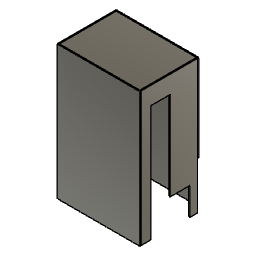
pc-case v8 (Autodesk Fusion 360 design; units mm, degrees)
Autodesk Fusion 360 part; units mm, degrees
sketch "Sketch1" plane through (0, 0, 0) normal (0, 1, 0) x (1, 0, 0) in component "Back"
  line L0 (0, 0) -> (210, 0)
  line L1 (210, 0) -> (210, -340)
  line L2 (210, -340) -> (0, -340)
  line L3 (0, -340) -> (0, 0)
  dimension "d1" = 210
  dimension "d2" = 340
  constraint horizontal L0
  constraint vertical L1
  constraint horizontal L2
  constraint vertical L3
  constraint coincident L0.start L3.end
  measures "d1" distance of L1.end L2.end
  measures "d2" distance of L0.start L2.end
extrude "Extrude1" add sketch "Sketch1" along normal blind 3 makes body 1 in component "Back"
sketch "Sketch1 (2)" plane through (0, 0, 0) normal (1, 0, 0) x (0, 1, 0) in component "right side"
  line L0 (2.986, 0.2323) -> (146.986, 0.2323)
  line L1 (146.986, 0.2323) -> (146.986, 310.2323)
  line L2 (146.986, 310.2323) -> (2.986, 310.2323)
  line L3 (2.986, 310.2323) -> (2.986, 0.2323)
  dimension "d5" = 310
  dimension "d6" = 144
  constraint horizontal L0
  constraint vertical L1
  constraint horizontal L2
  constraint vertical L3
  measures "d5" distance of L0.end L1.end
  measures "d6" distance of L0.start L0.end
extrude "Extrude1'" add sketch "Sketch1 (2)" along normal blind 3 separate body makes body 2 in component "right side"
sketch "Sketch1 (3)" plane through (0, 0, 0) normal (0, 0, 1) x (1, 0, 0) in component "top"
  line L0 (10, 145.6527) -> (214, 145.6527)
  line L1 (214, 145.6527) -> (214, 1.6527)
  line L2 (214, 1.6527) -> (10, 1.6527)
  line L3 (10, 1.6527) -> (10, 145.6527)
  dimension "d13" = 204
  dimension "d14" = 144
  constraint horizontal L0
  constraint vertical L1
  constraint horizontal L2
  constraint vertical L3
  measures "d13" distance of L0.start L0.end
  measures "d14" distance of L0.end L1.end
extrude "Extrude1''" add sketch "Sketch1 (3)" along normal blind 3 separate body makes body 3 in component "top"
sketch "Sketch1 (4)" plane through (0, 0, 0) normal (0, 1, 0) x (1, 0, 0) in component "front"
  line L0 (116.0218, -155.6494) -> (-93.9782, -155.6494)
  line L1 (-93.9782, -155.6494) -> (-93.9782, 169.3506)
  line L2 (-93.9782, 169.3506) -> (116.0218, 169.3506)
  line L3 (116.0218, 169.3506) -> (116.0218, -155.6494)
  dimension "d21" = 210
  dimension "d22" = 325
  constraint horizontal L0
  constraint vertical L1
  constraint horizontal L2
  constraint vertical L3
  measures "d21" distance of L0.start L0.end
  measures "d22" distance of L0.start L2.end
extrude "Extrude1'''" add sketch "Sketch1 (4)" along normal blind 3 separate body makes body 4 in component "front"
sketch "Sketch2" plane through (0, 0, 0) normal (1, 0, 0) x (0, 1, 0) in component "front"
sketch "Sketch1 (5)" plane through (0, 0, 0) normal (1, 0, 0) x (0, 1, 0) in component "left side"
  line L0 (-324, 340) -> (-180, 340)
  line L1 (-180, 340) -> (-180, 0)
  line L2 (-180, 0) -> (-200, 0)
  line L3 (-200, 0) -> (-200, 70)
  line L4 (-200, 70) -> (-250, 70)
  line L5 (-250, 70) -> (-250, 295)
  line L6 (-250, 295) -> (-299, 295)
  line L7 (-299, 295) -> (-299, 0)
  line L8 (-299, 0) -> (-324, 0)
  line L9 (-324, 0) -> (-324, 340)
  dimension "d29" = 144
  dimension "d30" = 340
  dimension "d31" = 295
  dimension "d32" = 25
  dimension "d33" = 20
  dimension "d34" = 70
  constraint horizontal L0
  constraint perpendicular L0 L1
  constraint perpendicular L1 L2
  constraint perpendicular L2 L3
  constraint perpendicular L1 L4
  constraint perpendicular L2 L5
  constraint perpendicular L5 L6
  constraint perpendicular L2 L7
  constraint perpendicular L7 L8
  constraint perpendicular L0 L9
  measures "d29" distance of L0.start L0.end
  measures "d30" distance of L0.end L1.end
  measures "d31" distance of L6.end L7.end
  measures "d32" distance of L7.end L8.end
  measures "d33" distance of L1.end L2.end
  measures "d34" distance of L2.end L3.end
extrude "Extrude1''''" add sketch "Sketch1 (5)" along normal blind 3 separate body makes body 5 in component "left side"
sketch "Sketch1 (6)" plane through (0, 0, 0) normal (0, 1, 0) x (1, 0, 0)
sketch "Sketch3" plane through (0, 3, 0) normal (0, 1, 0) x (-1, 0, 0) in component "front"
  line L0 (-116.0218, -169.3506) -> (93.9782, -169.3506)
  line L1 (93.9782, -169.3506) -> (93.9782, 155.6494)
  line L2 (93.9782, 155.6494) -> (-116.0218, 155.6494)
  line L3 (-116.0218, 155.6494) -> (-116.0218, -169.3506)
  line L4 (-116.0218, -169.3506) -> (-96.0218, -169.3506)
  line L5 (-96.0218, -169.3506) -> (-96.0218, -64.3506)
  line L6 (-96.0218, -64.3506) -> (-116.0218, -64.3506)
  line L7 (-116.0218, -64.3506) -> (-116.0218, -169.3506)
  dimension "d41" = 20
  dimension "d42" = 105
  constraint horizontal L4
  constraint vertical L5
  constraint horizontal L6
  constraint vertical L7
  constraint coincident L0.start L3.end
  measures "d41" distance of L5.end L6.end
  measures "d42" distance of L4.end L5.end
extrude "Extrude2" cut sketch "Sketch3" against normal blind 3 contours L0 L3 L4 L5 L6 L7 bodies 4 in component "front"
component "Back" placed x (1, 0, 0) y (0, 1, 0) z (0, 0, 1) at (7, -1.3473, -337)
component "right side" placed x (1, 0, 0) y (0, 1, 0) z (0, 0, 1) at (7, -1.3333, -307.2323)
component "top" placed x (1, 0, 0) y (0, 1, 0) z (0, 0, 1) at (0, 0, 0)
component "front" placed x (1, 0, 0) y (0, 1, 0) z (0, 0, 1) at (100.9782, 145.6527, -152.6494)
component "left side" placed x (1, 0, 0) y (0, 1, 0) z (0, 0, 1) at (214, 325.6527, -337)
